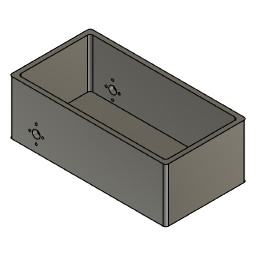
Micromouse_Base_3.0 v2 (Autodesk Fusion 360 design; units mm, degrees)
Autodesk Fusion 360 part; units mm, degrees
sketch "Skizze1" plane through (0, 0, 0) normal (0, 0, 1) x (1, 0, 0)
  line L0 (5, 0) -> (150, 0)
  line L1 (150, 0) -> (150, 75)
  line L2 (150, 75) -> (5, 75)
  line L3 (5, 75) -> (5, 0)
  constraint horizontal L0
  constraint vertical L1
  constraint horizontal L2
  constraint vertical L3
extrude "Extrusion1" add sketch "Skizze1" along normal blind 50
shell "Schale1" thickness 4.2 removed faces 1 at (53.3333, 50, 50)
fillet "Abrundung1" radius 2.5 1 edges at (5, 0, 25)
fillet "Abrundung2" radius 2.5 1 edges at (9.2, 4.2, 27.1)
fillet "Abrundung3" radius 2.5 1 edges at (9.2, 70.8, 27.1)
fillet "Abrundung4" radius 2.5 1 edges at (5, 75, 25)
fillet "Abrundung5" radius 2.5 1 edges at (150, 75, 25)
fillet "Abrundung6" radius 2.5 1 edges at (145.8, 70.8, 27.1)
fillet "Abrundung7" radius 2.5 1 edges at (145.8, 4.2, 27.1)
fillet "Abrundung8" radius 2.5 1 edges at (150, 0, 25)
sketch "Skizze2" plane through (0, 75, 0) normal (0, 1, 0) x (-1, 0, 0)
  line L0 (-147.5, 50) -> (-147.5, 0)
  line L1 (-147.5, 0) -> (-7.5, 0)
  line L2 (-7.5, 0) -> (-7.5, 50)
  line L3 (-7.5, 50) -> (-147.5, 50)
  circle A0 centre (-30, 7) radius 1
  dimension "d20" = 2
  measures "d20" diameter of A0
extrude "Extrusion2" cut sketch "Skizze2" against normal blind 300 contours A0
sketch "Skizze3" plane through (0, 75, 0) normal (0, 1, 0) x (-1, 0, 0)
  circle A0 centre (-30, 7) radius 1
  line L0 (-147.5, 50) -> (-147.5, 0)
  line L1 (-147.5, 0) -> (-7.5, 0)
  line L2 (-7.5, 0) -> (-7.5, 50)
  line L3 (-7.5, 50) -> (-147.5, 50)
  circle A1 centre (-30, 23) radius 1
  dimension "d23" = 2
  measures "d23" diameter of A1
extrude "Extrusion3" cut sketch "Skizze3" against normal blind 300 contours A1
sketch "Skizze4" plane through (0, 75, 0) normal (0, 1, 0) x (-1, 0, 0)
  circle A0 centre (-30, 23) radius 1
  circle A1 centre (-30, 7) radius 1
  line L0 (-147.5, 50) -> (-147.5, 0)
  line L1 (-147.5, 0) -> (-7.5, 0)
  line L2 (-7.5, 0) -> (-7.5, 50)
  line L3 (-7.5, 50) -> (-147.5, 50)
  circle A2 centre (-24, 15) radius 1
  circle A3 centre (-36, 15) radius 1
  dimension "d26" = 2
  dimension "d27" = 2
  measures "d26" diameter of A2
  measures "d27" diameter of A3
extrude "Extrusion4" cut sketch "Skizze4" against normal blind 300 contours A2
sketch "Skizze5" plane through (0, 75, 0) normal (0, 1, 0) x (-1, 0, 0)
  circle A0 centre (-24, 15) radius 1
  circle A1 centre (-30, 23) radius 1
  circle A2 centre (-30, 7) radius 1
  line L0 (-147.5, 50) -> (-147.5, 0)
  line L1 (-147.5, 0) -> (-7.5, 0)
  line L2 (-7.5, 0) -> (-7.5, 50)
  line L3 (-7.5, 50) -> (-147.5, 50)
  circle A3 centre (-36, 15) radius 1
  dimension "d30" = 2
  measures "d30" diameter of A3
extrude "Extrusion5" cut sketch "Skizze5" against normal blind 300 contours A3
sketch "Skizze6" plane through (0, 75, 0) normal (0, 1, 0) x (-1, 0, 0)
  circle A0 centre (-36, 15) radius 1
  circle A1 centre (-24, 15) radius 1
  circle A2 centre (-30, 23) radius 1
  circle A3 centre (-30, 7) radius 1
  line L0 (-147.5, 50) -> (-147.5, 0)
  line L1 (-147.5, 0) -> (-7.5, 0)
  line L2 (-7.5, 0) -> (-7.5, 50)
  line L3 (-7.5, 50) -> (-147.5, 50)
  circle A4 centre (-30, 15) radius 3.6
  dimension "d33" = 7.2
  measures "d33" diameter of A4
extrude "Extrusion6" cut sketch "Skizze6" against normal blind 300 contours A4
sketch "Skizze7" plane through (0, 0, 0) normal (0, 0, -1) x (1, 0, 0)
  arc A0 (150, -2.5) -> (147.5, 0) centre (147.5, -2.5) ccw
  line L0 (147.5, 0) -> (7.5, 0)
  arc A1 (7.5, 0) -> (5, -2.5) centre (7.5, -2.5) ccw
  line L1 (5, -2.5) -> (5, -72.5)
  arc A2 (5, -72.5) -> (7.5, -75) centre (7.5, -72.5) ccw
  line L2 (7.5, -75) -> (147.5, -75)
  arc A3 (147.5, -75) -> (150, -72.5) centre (147.5, -72.5) ccw
  line L3 (150, -72.5) -> (150, -2.5)
  line L4 (140, -29.5) -> (124, -29.5)
  line L5 (124, -29.5) -> (124, -45.5)
  line L6 (124, -45.5) -> (140, -45.5)
  line L7 (140, -45.5) -> (140, -29.5)
  constraint horizontal L4
  constraint vertical L5
  constraint horizontal L6
  constraint vertical L7
extrude "Extrusion7" cut sketch "Skizze7" against normal blind 2 contours L4 L5 L6 L7
